Autodesk Fusion 360 part; units mm, degrees
(part 2 of 7)
  spline S17 degree 5 poles (31.8463, -21.6348) (31.8387, -21.6182) (31.8236, -21.585) (31.8007, -21.5353) (31.7701, -21.4693) (31.7314, -21.387) (31.6925, -21.3049) (31.6532, -21.2232) (31.6135, -21.1418) (31.5736, -21.0606) (31.5333, -20.9798) (31.4926, -20.8992) (31.4516, -20.8189) (31.4103, -20.739) (31.3687, -20.6594) (31.3267, -20.58) (31.2844, -20.501) (31.2417, -20.4223) (31.1987, -20.3439) (31.1553, -20.2659) (31.1116, -20.1882) (31.0676, -20.1108) (31.0232, -20.0337) (30.9785, -19.957) (30.9334, -19.8806) (30.888, -19.8046) (30.8422, -19.7289) (30.796, -19.6536) (30.7496, -19.5787) (30.7027, -19.5041) (30.6555, -19.4299) (30.608, -19.356) (30.5601, -19.2825) (30.5118, -19.2094) (30.4631, -19.1368) (30.4141, -19.0645) (30.3647, -18.9925) (30.315, -18.921) (30.2649, -18.85) (30.2144, -18.7793) (30.1635, -18.709) (30.1123, -18.6392) (30.0606, -18.5699) (30.0086, -18.5009) (29.9561, -18.4325) (29.9033, -18.3645) (29.8501, -18.297) (29.7965, -18.2299) (29.7425, -18.1633) (29.6881, -18.0972) (29.6333, -18.0316) (29.578, -17.9666) (29.5222, -17.9021) (29.466, -17.8383) (29.4094, -17.775) (29.3523, -17.7122) (29.2948, -17.65) (29.2369, -17.5883) (29.1786, -17.5272) (29.1198, -17.4666) (29.0604, -17.4069) (29.0004, -17.348) (28.9396, -17.2901) (28.8782, -17.2332) (28.8162, -17.1772) (28.7537, -17.1217) (28.6909, -17.0668) (28.6278, -17.0123) (28.5642, -16.9585) (28.4998, -16.906) (28.434, -16.8556) (28.3799, -16.8175) (28.3382, -16.7905) (28.3099, -16.7732) (28.2957, -16.7647) knots -1 -1 -1 -1 -1 -1 -0.98571429 -0.97142857 -0.95714286 -0.94285714 -0.92857143 -0.91428571 -0.9 -0.88571429 -0.87142857 -0.85714286 -0.84285714 -0.82857143 -0.81428571 -0.8 -0.78571429 -0.77142857 -0.75714286 -0.74285714 -0.72857143 -0.71428571 -0.7 -0.68571429 -0.67142857 -0.65714286 -0.64285714 -0.62857143 -0.61428571 -0.6 -0.58571429 -0.57142857 -0.55714286 -0.54285714 -0.52857143 -0.51428571 -0.5 -0.48571429 -0.47142857 -0.45714286 -0.44285714 -0.42857143 -0.41428571 -0.4 -0.38571429 -0.37142857 -0.35714286 -0.34285714 -0.32857143 -0.31428571 -0.3 -0.28571429 -0.27142857 -0.25714286 -0.24285714 -0.22857143 -0.21428571 -0.2 -0.18571429 -0.17142857 -0.15714286 -0.14285714 -0.12857143 -0.11428571 -0.1 -0.08571429 -0.07142857 -0.05714286 -0.04285714 -0.02857143 -0.01428571 0 0 0 0 0 0
  line L17 (28.2957, -16.7647) -> (27.7863, -16.4626)
  arc A35 (27.1922, -14.356) -> (27.7863, -16.4626) centre (28.5961, -15.0972) ccw
  arc A36 (27.1922, -14.356) -> (27.5975, -13.5607) centre (0, 0) ccw
  arc A37 (29.6509, -12.8031) -> (27.5975, -13.5607) centre (29.0223, -14.2608) ccw
  line L18 (29.6509, -12.8031) -> (30.1947, -13.0376)
  spline S18 degree 5 poles (30.1947, -13.0376) (30.21, -13.0442) (30.2406, -13.0569) (30.2869, -13.0748) (30.3496, -13.0962) (30.429, -13.1197) (30.5094, -13.141) (30.5903, -13.1608) (30.6714, -13.1798) (30.7528, -13.1984) (30.8344, -13.2163) (30.9162, -13.2335) (30.9983, -13.2498) (31.0808, -13.2649) (31.1637, -13.2788) (31.247, -13.2917) (31.3305, -13.3037) (31.4142, -13.315) (31.4982, -13.3255) (31.5823, -13.3355) (31.6666, -13.3448) (31.7511, -13.3534) (31.8359, -13.3614) (31.9208, -13.3686) (32.0059, -13.3751) (32.0911, -13.3809) (32.1766, -13.3861) (32.2622, -13.3906) (32.348, -13.3946) (32.4339, -13.3979) (32.52, -13.4007) (32.6062, -13.4029) (32.6925, -13.4045) (32.779, -13.4055) (32.8656, -13.4059) (32.9523, -13.4058) (33.0392, -13.4051) (33.1262, -13.4038) (33.2132, -13.4021) (33.3004, -13.3997) (33.3877, -13.3969) (33.4751, -13.3935) (33.5626, -13.3896) (33.6502, -13.3852) (33.7379, -13.3803) (33.8257, -13.3748) (33.9136, -13.3689) (34.0016, -13.3624) (34.0896, -13.3555) (34.1778, -13.348) (34.266, -13.3401) (34.3542, -13.3317) (34.4426, -13.3228) (34.531, -13.3134) (34.6195, -13.3035) (34.7081, -13.2932) (34.7967, -13.2824) (34.8854, -13.2711) (34.9741, -13.2594) (35.063, -13.2472) (35.1518, -13.2345) (35.2407, -13.2214) (35.3297, -13.2078) (35.4187, -13.1938) (35.5078, -13.1793) (35.5969, -13.1644) (35.686, -13.1491) (35.7752, -13.1333) (35.8644, -13.117) (35.9537, -13.1003) (36.043, -13.0832) (36.1145, -13.0692) (36.1681, -13.0584) (36.2038, -13.0512) (36.2217, -13.0476) knots 0 0 0 0 0 0 0.01428571 0.02857143 0.04285714 0.05714286 0.07142857 0.08571429 0.1 0.11428571 0.12857143 0.14285714 0.15714286 0.17142857 0.18571429 0.2 0.21428571 0.22857143 0.24285714 0.25714286 0.27142857 0.28571429 0.3 0.31428571 0.32857143 0.34285714 0.35714286 0.37142857 0.38571429 0.4 0.41428571 0.42857143 0.44285714 0.45714286 0.47142857 0.48571429 0.5 0.51428571 0.52857143 0.54285714 0.55714286 0.57142857 0.58571429 0.6 0.61428571 0.62857143 0.64285714 0.65714286 0.67142857 0.68571429 0.7 0.71428571 0.72857143 0.74285714 0.75714286 0.77142857 0.78571429 0.8 0.81428571 0.82857143 0.84285714 0.85714286 0.87142857 0.88571429 0.9 0.91428571 0.92857143 0.94285714 0.95714286 0.97142857 0.98571429 1 1 1 1 1 1
  arc A38 (36.2217, -13.0476) -> (36.9731, -10.7349) centre (0, 0) ccw
  spline S19 degree 5 poles (36.9731, -10.7349) (36.9608, -10.7214) (36.9361, -10.6946) (36.8991, -10.6544) (36.8495, -10.601) (36.7873, -10.5347) (36.7249, -10.4687) (36.6623, -10.4031) (36.5994, -10.3379) (36.5363, -10.2731) (36.473, -10.2086) (36.4095, -10.1446) (36.3457, -10.0809) (36.2817, -10.0176) (36.2175, -9.9548) (36.153, -9.8923) (36.0883, -9.8302) (36.0235, -9.7686) (35.9583, -9.7073) (35.893, -9.6465) (35.8274, -9.5861) (35.7616, -9.5261) (35.6956, -9.4665) (35.6293, -9.4074) (35.5629, -9.3487) (35.4962, -9.2904) (35.4292, -9.2326) (35.3621, -9.1752) (35.2947, -9.1183) (35.2271, -9.0618) (35.1593, -9.0058) (35.0912, -8.9503) (35.023, -8.8952) (34.9545, -8.8406) (34.8857, -8.7865) (34.8168, -8.7329) (34.7476, -8.6798) (34.6782, -8.6271) (34.6086, -8.575) (34.5387, -8.5234) (34.4686, -8.4723) (34.3983, -8.4218) (34.3277, -8.3717) (34.257, -8.3223) (34.1859, -8.2734) (34.1147, -8.225) (34.0432, -8.1773) (33.9715, -8.13) (33.8996, -8.0834) (33.8274, -8.0373) (33.755, -7.9919) (33.6823, -7.9471) (33.6094, -7.9031) (33.5362, -7.8597) (33.4627, -7.817) (33.389, -7.775) (33.3151, -7.7336) (33.241, -7.6928) (33.1666, -7.6526) (33.092, -7.6133) (33.0171, -7.5748) (32.9418, -7.5373) (32.8662, -7.5011) (32.7902, -7.4659) (32.7139, -7.4318) (32.6373, -7.3983) (32.5606, -7.3655) (32.4838, -7.3332) (32.4067, -7.3017) (32.3292, -7.2716) (32.251, -7.244) (32.1878, -7.2245) (32.1398, -7.2117) (32.1076, -7.204) (32.0914, -7.2004) knots -1 -1 -1 -1 -1 -1 -0.98571429 -0.97142857 -0.95714286 -0.94285714 -0.92857143 -0.91428571 -0.9 -0.88571429 -0.87142857 -0.85714286 -0.84285714 -0.82857143 -0.81428571 -0.8 -0.78571429 -0.77142857 -0.75714286 -0.74285714 -0.72857143 -0.71428571 -0.7 -0.68571429 -0.67142857 -0.65714286 -0.64285714 -0.62857143 -0.61428571 -0.6 -0.58571429 -0.57142857 -0.55714286 -0.54285714 -0.52857143 -0.51428571 -0.5 -0.48571429 -0.47142857 -0.45714286 -0.44285714 -0.42857143 -0.41428571 -0.4 -0.38571429 -0.37142857 -0.35714286 -0.34285714 -0.32857143 -0.31428571 -0.3 -0.28571429 -0.27142857 -0.25714286 -0.24285714 -0.22857143 -0.21428571 -0.2 -0.18571429 -0.17142857 -0.15714286 -0.14285714 -0.12857143 -0.11428571 -0.1 -0.08571429 -0.07142857 -0.05714286 -0.04285714 -0.02857143 -0.01428571 0 0 0 0 0 0
  line L19 (32.0914, -7.2004) -> (31.5136, -7.0705)
  arc A39 (30.2976, -5.2505) -> (31.5136, -7.0705) centre (31.8618, -5.5216) ccw
  arc A40 (30.2976, -5.2505) -> (30.4372, -4.3689) centre (0, 0) ccw
  arc A41 (32.1561, -3.0138) -> (30.4372, -4.3689) centre (32.0086, -4.5945) ccw
  line L20 (32.1561, -3.0138) -> (32.7458, -3.0688)
  spline S20 degree 5 poles (32.7458, -3.0688) (32.7623, -3.0704) (32.7953, -3.073) (32.8449, -3.0757) (32.9111, -3.0767) (32.994, -3.0745) (33.0769, -3.0699) (33.16, -3.0638) (33.2431, -3.0568) (33.3262, -3.0493) (33.4093, -3.0411) (33.4924, -3.0322) (33.5756, -3.0223) (33.6587, -3.0111) (33.7419, -2.9988) (33.825, -2.9854) (33.9081, -2.971) (33.9913, -2.9558) (34.0744, -2.9399) (34.1575, -2.9233) (34.2405, -2.9061) (34.3236, -2.8882) (34.4066, -2.8696) (34.4896, -2.8502) (34.5725, -2.8301) (34.6554, -2.8093) (34.7383, -2.7878) (34.8211, -2.7657) (34.9039, -2.7429) (34.9867, -2.7195) (35.0694, -2.6956) (35.152, -2.671) (35.2346, -2.6459) (35.3172, -2.6201) (35.3997, -2.5937) (35.4821, -2.5668) (35.5645, -2.5393) (35.6469, -2.5113) (35.7291, -2.4827) (35.8113, -2.4535) (35.8935, -2.4238) (35.9756, -2.3936) (36.0576, -2.3629) (36.1395, -2.3316) (36.2214, -2.2998) (36.3032, -2.2675) (36.385, -2.2347) (36.4666, -2.2013) (36.5482, -2.1675) (36.6297, -2.1332) (36.7112, -2.0984) (36.7925, -2.0631) (36.8738, -2.0274) (36.955, -1.9911) (37.0361, -1.9544) (37.1172, -1.9172) (37.1981, -1.8795) (37.279, -1.8414) (37.3598, -1.8028) (37.4405, -1.7638) (37.5211, -1.7243) (37.6016, -1.6843) (37.682, -1.6439) (37.7623, -1.6031) (37.8425, -1.5618) (37.9227, -1.5201) (38.0027, -1.4779) (38.0826, -1.4353) (38.1625, -1.3923) (38.2422, -1.3489) (38.3218, -1.305) (38.3855, -1.2695) (38.4332, -1.2428) (38.4649, -1.2248) (38.4808, -1.2158) knots 0 0 0 0 0 0 0.01428571 0.02857143 0.04285714 0.05714286 0.07142857 0.08571429 0.1 0.11428571 0.12857143 0.14285714 0.15714286 0.17142857 0.18571429 0.2 0.21428571 0.22857143 0.24285714 0.25714286 0.27142857 0.28571429 0.3 0.31428571 0.32857143 0.34285714 0.35714286 0.37142857 0.38571429 0.4 0.41428571 0.42857143 0.44285714 0.45714286 0.47142857 0.48571429 0.5 0.51428571 0.52857143 0.54285714 0.55714286 0.57142857 0.58571429 0.6 0.61428571 0.62857143 0.64285714 0.65714286 0.67142857 0.68571429 0.7 0.71428571 0.72857143 0.74285714 0.75714286 0.77142857 0.78571429 0.8 0.81428571 0.82857143 0.84285714 0.85714286 0.87142857 0.88571429 0.9 0.91428571 0.92857143 0.94285714 0.95714286 0.97142857 0.98571429 1 1 1 1 1 1
  arc A42 (38.4808, -1.2158) -> (38.4808, 1.2158) centre (0, 0) ccw
  spline S21 degree 5 poles (38.4808, 1.2158) (38.4649, 1.2248) (38.4332, 1.2428) (38.3855, 1.2695) (38.3218, 1.305) (38.2422, 1.3489) (38.1625, 1.3923) (38.0826, 1.4353) (38.0027, 1.4779) (37.9227, 1.5201) (37.8425, 1.5618) (37.7623, 1.6031) (37.682, 1.6439) (37.6016, 1.6843) (37.5211, 1.7243) (37.4405, 1.7638) (37.3598, 1.8028) (37.279, 1.8414) (37.1981, 1.8795) (37.1172, 1.9172) (37.0361, 1.9544) (36.955, 1.9911) (36.8738, 2.0274) (36.7925, 2.0631) (36.7112, 2.0984) (36.6297, 2.1332) (36.5482, 2.1675) (36.4666, 2.2013) (36.385, 2.2347) (36.3032, 2.2675) (36.2214, 2.2998) (36.1395, 2.3316) (36.0576, 2.3629) (35.9756, 2.3936) (35.8935, 2.4238) (35.8113, 2.4535) (35.7291, 2.4827) (35.6469, 2.5113) (35.5645, 2.5393) (35.4821, 2.5668) (35.3997, 2.5937) (35.3172, 2.6201) (35.2346, 2.6459) (35.152, 2.671) (35.0694, 2.6956) (34.9867, 2.7195) (34.9039, 2.7429) (34.8211, 2.7657) (34.7383, 2.7878) (34.6554, 2.8093) (34.5725, 2.8301) (34.4896, 2.8502) (34.4066, 2.8696) (34.3236, 2.8882) (34.2405, 2.9061) (34.1575, 2.9233) (34.0744, 2.9399) (33.9913, 2.9558) (33.9081, 2.971) (33.825, 2.9854) (33.7419, 2.9988) (33.6587, 3.0111) (33.5756, 3.0223) (33.4924, 3.0322) (33.4093, 3.0411) (33.3262, 3.0493) (33.2431, 3.0568) (33.16, 3.0638) (33.0769, 3.0699) (32.994, 3.0745) (32.9111, 3.0767) (32.8449, 3.0757) (32.7953, 3.073) (32.7623, 3.0704) (32.7458, 3.0688) knots -1 -1 -1 -1 -1 -1 -0.98571429 -0.97142857 -0.95714286 -0.94285714 -0.92857143 -0.91428571 -0.9 -0.88571429 -0.87142857 -0.85714286 -0.84285714 -0.82857143 -0.81428571 -0.8 -0.78571429 -0.77142857 -0.75714286 -0.74285714 -0.72857143 -0.71428571 -0.7 -0.68571429 -0.67142857 -0.65714286 -0.64285714 -0.62857143 -0.61428571 -0.6 -0.58571429 -0.57142857 -0.55714286 -0.54285714 -0.52857143 -0.51428571 -0.5 -0.48571429 -0.47142857 -0.45714286 -0.44285714 -0.42857143 -0.41428571 -0.4 -0.38571429 -0.37142857 -0.35714286 -0.34285714 -0.32857143 -0.31428571 -0.3 -0.28571429 -0.27142857 -0.25714286 -0.24285714 -0.22857143 -0.21428571 -0.2 -0.18571429 -0.17142857 -0.15714286 -0.14285714 -0.12857143 -0.11428571 -0.1 -0.08571429 -0.07142857 -0.05714286 -0.04285714 -0.02857143 -0.01428571 0 0 0 0 0 0
  line L21 (32.7458, 3.0688) -> (32.1561, 3.0138)
  arc A43 (30.4372, 4.3689) -> (32.1561, 3.0138) centre (32.0086, 4.5945) ccw
  arc A44 (30.4372, 4.3689) -> (30.2976, 5.2505) centre (0, 0) ccw
  arc A45 (31.5136, 7.0705) -> (30.2976, 5.2505) centre (31.8618, 5.5216) ccw
  line L22 (31.5136, 7.0705) -> (32.0914, 7.2004)
  spline S22 degree 5 poles (32.0914, 7.2004) (32.1076, 7.204) (32.1398, 7.2117) (32.1878, 7.2245) (32.251, 7.244) (32.3292, 7.2716) (32.4067, 7.3017) (32.4838, 7.3332) (32.5606, 7.3655) (32.6373, 7.3983) (32.7139, 7.4318) (32.7902, 7.4659) (32.8662, 7.5011) (32.9418, 7.5373) (33.0171, 7.5748) (33.092, 7.6133) (33.1666, 7.6526) (33.241, 7.6928) (33.3151, 7.7336) (33.389, 7.775) (33.4627, 7.817) (33.5362, 7.8597) (33.6094, 7.9031) (33.6823, 7.9471) (33.755, 7.9919) (33.8274, 8.0373) (33.8996, 8.0834) (33.9715, 8.13) (34.0432, 8.1773) (34.1147, 8.225) (34.1859, 8.2734) (34.257, 8.3223) (34.3277, 8.3717) (34.3983, 8.4218) (34.4686, 8.4723) (34.5387, 8.5234) (34.6086, 8.575) (34.6782, 8.6271) (34.7476, 8.6798) (34.8168, 8.7329) (34.8857, 8.7865) (34.9545, 8.8406) (35.023, 8.8952) (35.0912, 8.9503) (35.1593, 9.0058) (35.2271, 9.0618) (35.2947, 9.1183) (35.3621, 9.1752) (35.4292, 9.2326) (35.4962, 9.2904) (35.5629, 9.3487) (35.6293, 9.4074) (35.6956, 9.4665) (35.7616, 9.5261) (35.8274, 9.5861) (35.893, 9.6465) (35.9583, 9.7073) (36.0235, 9.7686) (36.0883, 9.8302) (36.153, 9.8923) (36.2175, 9.9548) (36.2817, 10.0176) (36.3457, 10.0809) (36.4095, 10.1446) (36.473, 10.2086) (36.5363, 10.2731) (36.5994, 10.3379) (36.6623, 10.4031) (36.7249, 10.4687) (36.7873, 10.5347) (36.8495, 10.601) (36.8991, 10.6544) (36.9361, 10.6946) (36.9608, 10.7214) (36.9731, 10.7349) knots 0 0 0 0 0 0 0.01428571 0.02857143 0.04285714 0.05714286 0.07142857 0.08571429 0.1 0.11428571 0.12857143 0.14285714 0.15714286 0.17142857 0.18571429 0.2 0.21428571 0.22857143 0.24285714 0.25714286 0.27142857 0.28571429 0.3 0.31428571 0.32857143 0.34285714 0.35714286 0.37142857 0.38571429 0.4 0.41428571 0.42857143 0.44285714 0.45714286 0.47142857 0.48571429 0.5 0.51428571 0.52857143 0.54285714 0.55714286 0.57142857 0.58571429 0.6 0.61428571 0.62857143 0.64285714 0.65714286 0.67142857 0.68571429 0.7 0.71428571 0.72857143 0.74285714 0.75714286 0.77142857 0.78571429 0.8 0.81428571 0.82857143 0.84285714 0.85714286 0.87142857 0.88571429 0.9 0.91428571 0.92857143 0.94285714 0.95714286 0.97142857 0.98571429 1 1 1 1 1 1
  arc A46 (36.9731, 10.7349) -> (36.2217, 13.0476) centre (0, 0) ccw
  spline S23 degree 5 poles (36.2217, 13.0476) (36.2038, 13.0512) (36.1681, 13.0584) (36.1145, 13.0692) (36.043, 13.0832) (35.9537, 13.1003) (35.8644, 13.117) (35.7752, 13.1333) (35.686, 13.1491) (35.5969, 13.1644) (35.5078, 13.1793) (35.4187, 13.1938) (35.3297, 13.2078) (35.2407, 13.2214) (35.1518, 13.2345) (35.063, 13.2472) (34.9741, 13.2594) (34.8854, 13.2711) (34.7967, 13.2824) (34.7081, 13.2932) (34.6195, 13.3035) (34.531, 13.3134) (34.4426, 13.3228) (34.3542, 13.3317) (34.266, 13.3401) (34.1778, 13.348) (34.0896, 13.3555) (34.0016, 13.3624) (33.9136, 13.3689) (33.8257, 13.3748) (33.7379, 13.3803) (33.6502, 13.3852) (33.5626, 13.3896) (33.4751, 13.3935) (33.3877, 13.3969) (33.3004, 13.3997) (33.2132, 13.4021) (33.1262, 13.4038) (33.0392, 13.4051) (32.9523, 13.4058) (32.8656, 13.4059) (32.779, 13.4055) (32.6925, 13.4045) (32.6062, 13.4029) (32.52, 13.4007) (32.4339, 13.3979) (32.348, 13.3946) (32.2622, 13.3906) (32.1766, 13.3861) (32.0911, 13.3809) (32.0059, 13.3751) (31.9208, 13.3686) (31.8359, 13.3614) (31.7511, 13.3534) (31.6666, 13.3448) (31.5823, 13.3355) (31.4982, 13.3255) (31.4142, 13.315) (31.3305, 13.3037) (31.247, 13.2917) (31.1637, 13.2788) (31.0808, 13.2649) (30.9983, 13.2498) (30.9162, 13.2335) (30.8344, 13.2163) (30.7528, 13.1984) (30.6714, 13.1798) (30.5903, 13.1608) (30.5094, 13.141) (30.429, 13.1197) (30.3496, 13.0962) (30.2869, 13.0748) (30.2406, 13.0569) (30.21, 13.0442) (30.1947, 13.0376) knots -1 -1 -1 -1 -1 -1 -0.98571429 -0.97142857 -0.95714286 -0.94285714 -0.92857143 -0.91428571 -0.9 -0.88571429 -0.87142857 -0.85714286 -0.84285714 -0.82857143 -0.81428571 -0.8 -0.78571429 -0.77142857 -0.75714286 -0.74285714 -0.72857143 -0.71428571 -0.7 -0.68571429 -0.67142857 -0.65714286 -0.64285714 -0.62857143 -0.61428571 -0.6 -0.58571429 -0.57142857 -0.55714286 -0.54285714 -0.52857143 -0.51428571 -0.5 -0.48571429 -0.47142857 -0.45714286 -0.44285714 -0.42857143 -0.41428571 -0.4 -0.38571429 -0.37142857 -0.35714286 -0.34285714 -0.32857143 -0.31428571 -0.3 -0.28571429 -0.27142857 -0.25714286 -0.24285714 -0.22857143 -0.21428571 -0.2 -0.18571429 -0.17142857 -0.15714286 -0.14285714 -0.12857143 -0.11428571 -0.1 -0.08571429 -0.07142857 -0.05714286 -0.04285714 -0.02857143 -0.01428571 0 0 0 0 0 0
  line L23 (30.1947, 13.0376) -> (29.6509, 12.8031)
  arc A47 (27.5975, 13.5607) -> (29.6509, 12.8031) centre (29.0223, 14.2608) ccw
  arc A48 (27.5975, 13.5607) -> (27.1922, 14.356) centre (0, 0) ccw
  arc A49 (27.7863, 16.4626) -> (27.1922, 14.356) centre (28.5961, 15.0972) ccw
  line L24 (27.7863, 16.4626) -> (28.2957, 16.7647)
  spline S24 degree 5 poles (28.2957, 16.7647) (28.3099, 16.7732) (28.3382, 16.7905) (28.3799, 16.8175) (28.434, 16.8556) (28.4998, 16.906) (28.5642, 16.9585) (28.6278, 17.0123) (28.6909, 17.0668) (28.7537, 17.1217) (28.8162, 17.1772) (28.8782, 17.2332) (28.9396, 17.2901) (29.0004, 17.348) (29.0604, 17.4069) (29.1198, 17.4666) (29.1786, 17.5272) (29.2369, 17.5883) (29.2948, 17.65) (29.3523, 17.7122) (29.4094, 17.775) (29.466, 17.8383) (29.5222, 17.9021) (29.578, 17.9666) (29.6333, 18.0316) (29.6881, 18.0972) (29.7425, 18.1633) (29.7965, 18.2299) (29.8501, 18.297) (29.9033, 18.3645) (29.9561, 18.4325) (30.0086, 18.5009) (30.0606, 18.5699) (30.1123, 18.6392) (30.1635, 18.709) (30.2144, 18.7793) (30.2649, 18.85) (30.315, 18.921) (30.3647, 18.9925) (30.4141, 19.0645) (30.4631, 19.1368) (30.5118, 19.2094) (30.5601, 19.2825) (30.608, 19.356) (30.6555, 19.4299) (30.7027, 19.5041) (30.7496, 19.5787) (30.796, 19.6536) (30.8422, 19.7289) (30.888, 19.8046) (30.9334, 19.8806) (30.9785, 19.957) (31.0232, 20.0337) (31.0676, 20.1108) (31.1116, 20.1882) (31.1553, 20.2659) (31.1987, 20.3439) (31.2417, 20.4223) (31.2844, 20.501) (31.3267, 20.58) (31.3687, 20.6594) (31.4103, 20.739) (31.4516, 20.8189) (31.4926, 20.8992) (31.5333, 20.9798) (31.5736, 21.0606) (31.6135, 21.1418) (31.6532, 21.2232) (31.6925, 21.3049) (31.7314, 21.387) (31.7701, 21.4693) (31.8007, 21.5353) (31.8236, 21.585) (31.8387, 21.6182) (31.8463, 21.6348) knots 0 0 0 0 0 0 0.01428571 0.02857143 0.04285714 0.05714286 0.07142857 0.08571429 0.1 0.11428571 0.12857143 0.14285714 0.15714286 0.17142857 0.18571429 0.2 0.21428571 0.22857143 0.24285714 0.25714286 0.27142857 0.28571429 0.3 0.31428571 0.32857143 0.34285714 0.35714286 0.37142857 0.38571429 0.4 0.41428571 0.42857143 0.44285714 0.45714286 0.47142857 0.48571429 0.5 0.51428571 0.52857143 0.54285714 0.55714286 0.57142857 0.58571429 0.6 0.61428571 0.62857143 0.64285714 0.65714286 0.67142857 0.68571429 0.7 0.71428571 0.72857143 0.74285714 0.75714286 0.77142857 0.78571429 0.8 0.81428571 0.82857143 0.84285714 0.85714286 0.87142857 0.88571429 0.9 0.91428571 0.92857143 0.94285714 0.95714286 0.97142857 0.98571429 1 1 1 1 1 1
  arc A50 (31.8463, 21.6348) -> (30.417, 23.6021) centre (0, 0) ccw
  spline S25 degree 5 poles (30.417, 23.6021) (30.3988, 23.6) (30.3626, 23.5959) (30.3083, 23.5895) (30.236, 23.5808) (30.1458, 23.5695) (30.0557, 23.5577) (29.9658, 23.5456) (29.8761, 23.5331) (29.7866, 23.5201) (29.6972, 23.5068) (29.6081, 23.493) (29.5191, 23.4789) (29.4303, 23.4643) (29.3417, 23.4493) (29.2532, 23.4339) (29.165, 23.418) (29.077, 23.4018) (28.9892, 23.3851) (28.9015, 23.368) (28.8141, 23.3504) (28.7269, 23.3325) (28.6399, 23.3141) (28.5531, 23.2952) (28.4666, 23.2759) (28.3802, 23.2562) (28.2941, 23.2361) (28.2082, 23.2155) (28.1226, 23.1944) (28.0371, 23.1729) (27.952, 23.151) (27.867, 23.1286) (27.7824, 23.1057) (27.6979, 23.0824) (27.6138, 23.0586) (27.5298, 23.0343) (27.4462, 23.0096) (27.3628, 22.9844) (27.2797, 22.9587) (27.1969, 22.9325) (27.1144, 22.9058) (27.0322, 22.8786) (26.9502, 22.8509) (26.8686, 22.8227) (26.7873, 22.794) (26.7063, 22.7648) (26.6256, 22.7351) (26.5453, 22.7048) (26.4652, 22.674) (26.3856, 22.6427) (26.3062, 22.6108) (26.2273, 22.5783) (26.1488, 22.5452) (26.0707, 22.5115) (25.993, 22.4772) (25.9157, 22.4423) (25.8387, 22.4068) (25.7622, 22.3708) (25.686, 22.3343) (25.6103, 22.297) (25.5351, 22.259) (25.4606, 22.2202) (25.3867, 22.1803) (25.3136, 22.1395) (25.2411, 22.0978) (25.1691, 22.0555) (25.0975, 22.0128) (25.0261, 21.9696) (24.9554, 21.9257) (24.8855, 21.8807) (24.8172, 21.8337) (24.7642, 21.794) (24.7257, 21.7627) (24.7005, 21.7412) (24.6881, 21.7302) knots -1 -1 -1 -1 -1 -1 -0.98571429 -0.97142857 -0.95714286 -0.94285714 -0.92857143 -0.91428571 -0.9 -0.88571429 -0.87142857 -0.85714286 -0.84285714 -0.82857143 -0.81428571 -0.8 -0.78571429 -0.77142857 -0.75714286 -0.74285714 -0.72857143 -0.71428571 -0.7 -0.68571429 -0.67142857 -0.65714286 -0.64285714 -0.62857143 -0.61428571 -0.6 -0.58571429 -0.57142857 -0.55714286 -0.54285714 -0.52857143 -0.51428571 -0.5 -0.48571429 -0.47142857 -0.45714286 -0.44285714 -0.42857143 -0.41428571 -0.4 -0.38571429 -0.37142857 -0.35714286 -0.34285714 -0.32857143 -0.31428571 -0.3 -0.28571429 -0.27142857 -0.25714286 -0.24285714 -0.22857143 -0.21428571 -0.2 -0.18571429 -0.17142857 -0.15714286 -0.14285714 -0.12857143 -0.11428571 -0.1 -0.08571429 -0.07142857 -0.05714286 -0.04285714 -0.02857143 -0.01428571 0 0 0 0 0 0
  line L25 (24.6881, 21.7302) -> (24.2433, 21.3391)
  arc A51 (22.0563, 21.4251) -> (24.2433, 21.3391) centre (23.195, 22.5312) ccw
  arc A52 (22.0563, 21.4251) -> (21.4251, 22.0563) centre (0, 0) ccw
  arc A53 (21.3391, 24.2433) -> (21.4251, 22.0563) centre (22.5312, 23.195) ccw
  line L26 (21.3391, 24.2433) -> (21.7302, 24.6881)
  spline S26 degree 5 poles (21.7302, 24.6881) (21.7412, 24.7005) (21.7627, 24.7257) (21.794, 24.7642) (21.8337, 24.8172) (21.8807, 24.8855) (21.9257, 24.9554) (21.9696, 25.0261) (22.0128, 25.0975) (22.0555, 25.1691) (22.0978, 25.2411) (22.1395, 25.3136) (22.1803, 25.3867) (22.2202, 25.4606) (22.259, 25.5351) (22.297, 25.6103) (22.3343, 25.686) (22.3708, 25.7622) (22.4068, 25.8387) (22.4423, 25.9157) (22.4772, 25.993) (22.5115, 26.0707) (22.5452, 26.1488) (22.5783, 26.2273) (22.6108, 26.3062) (22.6427, 26.3856) (22.674, 26.4652) (22.7048, 26.5453) (22.7351, 26.6256) (22.7648, 26.7063) (22.794, 26.7873) (22.8227, 26.8686) (22.8509, 26.9502) (22.8786, 27.0322) (22.9058, 27.1144) (22.9325, 27.1969) (22.9587, 27.2797) (22.9844, 27.3628) (23.0096, 27.4462) (23.0343, 27.5298) (23.0586, 27.6138) (23.0824, 27.6979) (23.1057, 27.7824) (23.1286, 27.867) (23.151, 27.952) (23.1729, 28.0371) (23.1944, 28.1226) (23.2155, 28.2082) (23.2361, 28.2941) (23.2562, 28.3802) (23.2759, 28.4666) (23.2952, 28.5531) (23.3141, 28.6399) (23.3325, 28.7269) (23.3504, 28.8141) (23.368, 28.9015) (23.3851, 28.9892) (23.4018, 29.077) (23.418, 29.165) (23.4339, 29.2532) (23.4493, 29.3417) (23.4643, 29.4303) (23.4789, 29.5191) (23.493, 29.6081) (23.5068, 29.6972) (23.5201, 29.7866) (23.5331, 29.8761) (23.5456, 29.9658) (23.5577, 30.0557) (23.5695, 30.1458) (23.5808, 30.236) (23.5895, 30.3083) (23.5959, 30.3626) (23.6, 30.3988) (23.6021, 30.417) knots 0 0 0 0 0 0 0.01428571 0.02857143 0.04285714 0.05714286 0.07142857 0.08571429 0.1 0.11428571 0.12857143 0.14285714 0.15714286 0.17142857 0.18571429 0.2 0.21428571 0.22857143 0.24285714 0.25714286 0.27142857 0.28571429 0.3 0.31428571 0.32857143 0.34285714 0.35714286 0.37142857 0.38571429 0.4 0.41428571 0.42857143 0.44285714 0.45714286 0.47142857 0.48571429 0.5 0.51428571 0.52857143 0.54285714 0.55714286 0.57142857 0.58571429 0.6 0.61428571 0.62857143 0.64285714 0.65714286 0.67142857 0.68571429 0.7 0.71428571 0.72857143 0.74285714 0.75714286 0.77142857 0.78571429 0.8 0.81428571 0.82857143 0.84285714 0.85714286 0.87142857 0.88571429 0.9 0.91428571 0.92857143 0.94285714 0.95714286 0.97142857 0.98571429 1 1 1 1 1 1
  arc A54 (23.6021, 30.417) -> (21.6348, 31.8463) centre (0, 0) ccw
  spline S27 degree 5 poles (21.6348, 31.8463) (21.6182, 31.8387) (21.585, 31.8236) (21.5353, 31.8007) (21.4693, 31.7701) (21.387, 31.7314) (21.3049, 31.6925) (21.2232, 31.6532) (21.1418, 31.6135) (21.0606, 31.5736) (20.9798, 31.5333) (20.8992, 31.4926) (20.8189, 31.4516) (20.739, 31.4103) (20.6594, 31.3687) (20.58, 31.3267) (20.501, 31.2844) (20.4223, 31.2417) (20.3439, 31.1987) (20.2659, 31.1553) (20.1882, 31.1116) (20.1108, 31.0676) (20.0337, 31.0232) (19.957, 30.9785) (19.8806, 30.9334) (19.8046, 30.888) (19.7289, 30.8422) (19.6536, 30.796) (19.5787, 30.7496) (19.5041, 30.7027) (19.4299, 30.6555) (19.356, 30.608) (19.2825, 30.5601) (19.2094, 30.5118) (19.1368, 30.4631) (19.0645, 30.4141) (18.9925, 30.3647) (18.921, 30.315) (18.85, 30.2649) (18.7793, 30.2144) (18.709, 30.1635) (18.6392, 30.1123) (18.5699, 30.0606) (18.5009, 30.0086) (18.4325, 29.9561) (18.3645, 29.9033) (18.297, 29.8501) (18.2299, 29.7965) (18.1633, 29.7425) (18.0972, 29.6881) (18.0316, 29.6333) (17.9666, 29.578) (17.9021, 29.5222) (17.8383, 29.466) (17.775, 29.4094) (17.7122, 29.3523) (17.65, 29.2948) (17.5883, 29.2369) (17.5272, 29.1786) (17.4666, 29.1198) (17.4069, 29.0604) (17.348, 29.0004) (17.2901, 28.9396) (17.2332, 28.8782) (17.1772, 28.8162) (17.1217, 28.7537) (17.0668, 28.6909) (17.0123, 28.6278) (16.9585, 28.5642) (16.906, 28.4998) (16.8556, 28.434) (16.8175, 28.3799) (16.7905, 28.3382) (16.7732, 28.3099) (16.7647, 28.2957) knots -1 -1 -1 -1 -1 -1 -0.98571429 -0.97142857 -0.95714286 -0.94285714 -0.92857143 -0.91428571 -0.9 -0.88571429 -0.87142857 -0.85714286 -0.84285714 -0.82857143 -0.81428571 -0.8 -0.78571429 -0.77142857 -0.75714286 -0.74285714 -0.72857143 -0.71428571 -0.7 -0.68571429 -0.67142857 -0.65714286 -0.64285714 -0.62857143 -0.61428571 -0.6 -0.58571429 -0.57142857 -0.55714286 -0.54285714 -0.52857143 -0.51428571 -0.5 -0.48571429 -0.47142857 -0.45714286 -0.44285714 -0.42857143 -0.41428571 -0.4 -0.38571429 -0.37142857 -0.35714286 -0.34285714 -0.32857143 -0.31428571 -0.3 -0.28571429 -0.27142857 -0.25714286 -0.24285714 -0.22857143 -0.21428571 -0.2 -0.18571429 -0.17142857 -0.15714286 -0.14285714 -0.12857143 -0.11428571 -0.1 -0.08571429 -0.07142857 -0.05714286 -0.04285714 -0.02857143 -0.01428571 0 0 0 0 0 0
  line L27 (16.7647, 28.2957) -> (16.4626, 27.7863)
  arc A55 (14.356, 27.1922) -> (16.4626, 27.7863) centre (15.0972, 28.5961) ccw
  arc A56 (14.356, 27.1922) -> (13.5607, 27.5975) centre (0, 0) ccw
  arc A57 (12.8031, 29.6509) -> (13.5607, 27.5975) centre (14.2608, 29.0223) ccw
  line L28 (12.8031, 29.6509) -> (13.0376, 30.1947)
  spline S28 degree 5 poles (13.0376, 30.1947) (13.0442, 30.21) (13.0569, 30.2406) (13.0748, 30.2869) (13.0962, 30.3496) (13.1197, 30.429) (13.141, 30.5094) (13.1608, 30.5903) (13.1798, 30.6714) (13.1984, 30.7528) (13.2163, 30.8344) (13.2335, 30.9162) (13.2498, 30.9983) (13.2649, 31.0808) (13.2788, 31.1637) (13.2917, 31.247) (13.3037, 31.3305) (13.315, 31.4142) (13.3255, 31.4982) (13.3355, 31.5823) (13.3448, 31.6666) (13.3534, 31.7511) (13.3614, 31.8359) (13.3686, 31.9208) (13.3751, 32.0059) (13.3809, 32.0911) (13.3861, 32.1766) (13.3906, 32.2622) (13.3946, 32.348) (13.3979, 32.4339) (13.4007, 32.52) (13.4029, 32.6062) (13.4045, 32.6925) (13.4055, 32.779) (13.4059, 32.8656) (13.4058, 32.9523) (13.4051, 33.0392) (13.4038, 33.1262) (13.4021, 33.2132) (13.3997, 33.3004) (13.3969, 33.3877) (13.3935, 33.4751) (13.3896, 33.5626) (13.3852, 33.6502) (13.3803, 33.7379) (13.3748, 33.8257) (13.3689, 33.9136) (13.3624, 34.0016) (13.3555, 34.0896) (13.348, 34.1778) (13.3401, 34.266) (13.3317, 34.3542) (13.3228, 34.4426) (13.3134, 34.531) (13.3035, 34.6195) (13.2932, 34.7081) (13.2824, 34.7967) (13.2711, 34.8854) (13.2594, 34.9741) (13.2472, 35.063) (13.2345, 35.1518) (13.2214, 35.2407) (13.2078, 35.3297) (13.1938, 35.4187) (13.1793, 35.5078) (13.1644, 35.5969) (13.1491, 35.686) (13.1333, 35.7752) (13.117, 35.8644) (13.1003, 35.9537) (13.0832, 36.043) (13.0692, 36.1145) (13.0584, 36.1681) (13.0512, 36.2038) (13.0476, 36.2217) knots 0 0 0 0 0 0 0.01428571 0.02857143 0.04285714 0.05714286 0.07142857 0.08571429 0.1 0.11428571 0.12857143 0.14285714 0.15714286 0.17142857 0.18571429 0.2 0.21428571 0.22857143 0.24285714 0.25714286 0.27142857 0.28571429 0.3 0.31428571 0.32857143 0.34285714 0.35714286 0.37142857 0.38571429 0.4 0.41428571 0.42857143 0.44285714 0.45714286 0.47142857 0.48571429 0.5 0.51428571 0.52857143 0.54285714 0.55714286 0.57142857 0.58571429 0.6 0.61428571 0.62857143 0.64285714 0.65714286 0.67142857 0.68571429 0.7 0.71428571 0.72857143 0.74285714 0.75714286 0.77142857 0.78571429 0.8 0.81428571 0.82857143 0.84285714 0.85714286 0.87142857 0.88571429 0.9 0.91428571 0.92857143 0.94285714 0.95714286 0.97142857 0.98571429 1 1 1 1 1 1
  arc A58 (13.0476, 36.2217) -> (10.7349, 36.9731) centre (0, 0) ccw
  spline S29 degree 5 poles (10.7349, 36.9731) (10.7214, 36.9608) (10.6946, 36.9361) (10.6544, 36.8991) (10.601, 36.8495) (10.5347, 36.7873) (10.4687, 36.7249) (10.4031, 36.6623) (10.3379, 36.5994) (10.2731, 36.5363) (10.2086, 36.473) (10.1446, 36.4095) (10.0809, 36.3457) (10.0176, 36.2817) (9.9548, 36.2175) (9.8923, 36.153) (9.8302, 36.0883) (9.7686, 36.0235) (9.7073, 35.9583) (9.6465, 35.893) (9.5861, 35.8274) (9.5261, 35.7616) (9.4665, 35.6956) (9.4074, 35.6293) (9.3487, 35.5629) (9.2904, 35.4962) (9.2326, 35.4292) (9.1752, 35.3621) (9.1183, 35.2947) (9.0618, 35.2271) (9.0058, 35.1593) (8.9503, 35.0912) (8.8952, 35.023) (8.8406, 34.9545) (8.7865, 34.8857) (8.7329, 34.8168) (8.6798, 34.7476) (8.6271, 34.6782) (8.575, 34.6086) (8.5234, 34.5387) (8.4723, 34.4686) (8.4218, 34.3983) (8.3717, 34.3277) (8.3223, 34.257) (8.2734, 34.1859) (8.225, 34.1147) (8.1773, 34.0432) (8.13, 33.9715) (8.0834, 33.8996) (8.0373, 33.8274) (7.9919, 33.755) (7.9471, 33.6823) (7.9031, 33.6094) (7.8597, 33.5362) (7.817, 33.4627) (7.775, 33.389) (7.7336, 33.3151) (7.6928, 33.241) (7.6526, 33.1666) (7.6133, 33.092) (7.5748, 33.0171) (7.5373, 32.9418) (7.5011, 32.8662) (7.4659, 32.7902) (7.4318, 32.7139) (7.3983, 32.6373) (7.3655, 32.5606) (7.3332, 32.4838) (7.3017, 32.4067) (7.2716, 32.3292) (7.244, 32.251) (7.2245, 32.1878) (7.2117, 32.1398) (7.204, 32.1076) (7.2004, 32.0914) knots -1 -1 -1 -1 -1 -1 -0.98571429 -0.97142857 -0.95714286 -0.94285714 -0.92857143 -0.91428571 -0.9 -0.88571429 -0.87142857 -0.85714286 -0.84285714 -0.82857143 -0.81428571 -0.8 -0.78571429 -0.77142857 -0.75714286 -0.74285714 -0.72857143 -0.71428571 -0.7 -0.68571429 -0.67142857 -0.65714286 -0.64285714 -0.62857143 -0.61428571 -0.6 -0.58571429 -0.57142857 -0.55714286 -0.54285714 -0.52857143 -0.51428571 -0.5 -0.48571429 -0.47142857 -0.45714286 -0.44285714 -0.42857143 -0.41428571 -0.4 -0.38571429 -0.37142857 -0.35714286 -0.34285714 -0.32857143 -0.31428571 -0.3 -0.28571429 -0.27142857 -0.25714286 -0.24285714 -0.22857143 -0.21428571 -0.2 -0.18571429 -0.17142857 -0.15714286 -0.14285714 -0.12857143 -0.11428571 -0.1 -0.08571429 -0.07142857 -0.05714286 -0.04285714 -0.02857143 -0.01428571 0 0 0 0 0 0
  line L29 (7.2004, 32.0914) -> (7.0705, 31.5136)
  arc A59 (5.2505, 30.2976) -> (7.0705, 31.5136) centre (5.5216, 31.8618) ccw
  arc A60 (5.2505, 30.2976) -> (4.3689, 30.4372) centre (0, 0) ccw
  arc A61 (3.0138, 32.1561) -> (4.3689, 30.4372) centre (4.5945, 32.0086) ccw
  line L30 (3.0138, 32.1561) -> (3.0688, 32.7458)
  spline S30 degree 5 poles (3.0688, 32.7458) (3.0704, 32.7623) (3.073, 32.7953) (3.0757, 32.8449) (3.0767, 32.9111) (3.0745, 32.994) (3.0699, 33.0769) (3.0638, 33.16) (3.0568, 33.2431) (3.0493, 33.3262) (3.0411, 33.4093) (3.0322, 33.4924) (3.0223, 33.5756) (3.0111, 33.6587) (2.9988, 33.7419) (2.9854, 33.825) (2.971, 33.9081) (2.9558, 33.9913) (2.9399, 34.0744) (2.9233, 34.1575) (2.9061, 34.2405) (2.8882, 34.3236) (2.8696, 34.4066) (2.8502, 34.4896) (2.8301, 34.5725) (2.8093, 34.6554) (2.7878, 34.7383) (2.7657, 34.8211) (2.7429, 34.9039) (2.7195, 34.9867) (2.6956, 35.0694) (2.671, 35.152) (2.6459, 35.2346) (2.6201, 35.3172) (2.5937, 35.3997) (2.5668, 35.4821) (2.5393, 35.5645) (2.5113, 35.6469) (2.4827, 35.7291) (2.4535, 35.8113) (2.4238, 35.8935) (2.3936, 35.9756) (2.3629, 36.0576) (2.3316, 36.1395) (2.2998, 36.2214) (2.2675, 36.3032) (2.2347, 36.385) (2.2013, 36.4666) (2.1675, 36.5482) (2.1332, 36.6297) (2.0984, 36.7112) (2.0631, 36.7925) (2.0274, 36.8738) (1.9911, 36.955) (1.9544, 37.0361) (1.9172, 37.1172) (1.8795, 37.1981) (1.8414, 37.279) (1.8028, 37.3598) (1.7638, 37.4405) (1.7243, 37.5211) (1.6843, 37.6016) (1.6439, 37.682) (1.6031, 37.7623) (1.5618, 37.8425) (1.5201, 37.9227) (1.4779, 38.0027) (1.4353, 38.0826) (1.3923, 38.1625) (1.3489, 38.2422) (1.305, 38.3218) (1.2695, 38.3855) (1.2428, 38.4332) (1.2248, 38.4649) (1.2158, 38.4808) knots 0 0 0 0 0 0 0.01428571 0.02857143 0.04285714 0.05714286 0.07142857 0.08571429 0.1 0.11428571 0.12857143 0.14285714 0.15714286 0.17142857 0.18571429 0.2 0.21428571 0.22857143 0.24285714 0.25714286 0.27142857 0.28571429 0.3 0.31428571 0.32857143 0.34285714 0.35714286 0.37142857 0.38571429 0.4 0.41428571 0.42857143 0.44285714 0.45714286 0.47142857 0.48571429 0.5 0.51428571 0.52857143 0.54285714 0.55714286 0.57142857 0.58571429 0.6 0.61428571 0.62857143 0.64285714 0.65714286 0.67142857 0.68571429 0.7 0.71428571 0.72857143 0.74285714 0.75714286 0.77142857 0.78571429 0.8 0.81428571 0.82857143 0.84285714 0.85714286 0.87142857 0.88571429 0.9 0.91428571 0.92857143 0.94285714 0.95714286 0.97142857 0.98571429 1 1 1 1 1 1
  arc A62 (1.2158, 38.4808) -> (-1.2158, 38.4808) centre (0, 0) ccw
  spline S31 degree 5 poles (-1.2158, 38.4808) (-1.2248, 38.4649) (-1.2428, 38.4332) (-1.2695, 38.3855) (-1.305, 38.3218) (-1.3489, 38.2422) (-1.3923, 38.1625) (-1.4353, 38.0826) (-1.4779, 38.0027) (-1.5201, 37.9227) (-1.5618, 37.8425) (-1.6031, 37.7623) (-1.6439, 37.682) (-1.6843, 37.6016) (-1.7243, 37.5211) (-1.7638, 37.4405) (-1.8028, 37.3598) (-1.8414, 37.279) (-1.8795, 37.1981) (-1.9172, 37.1172) (-1.9544, 37.0361) (-1.9911, 36.955) (-2.0274, 36.8738) (-2.0631, 36.7925) (-2.0984, 36.7112) (-2.1332, 36.6297) (-2.1675, 36.5482) (-2.2013, 36.4666) (-2.2347, 36.385) (-2.2675, 36.3032) (-2.2998, 36.2214) (-2.3316, 36.1395) (-2.3629, 36.0576) (-2.3936, 35.9756) (-2.4238, 35.8935) (-2.4535, 35.8113) (-2.4827, 35.7291) (-2.5113, 35.6469) (-2.5393, 35.5645) (-2.5668, 35.4821) (-2.5937, 35.3997) (-2.6201, 35.3172) (-2.6459, 35.2346) (-2.671, 35.152) (-2.6956, 35.0694) (-2.7195, 34.9867) (-2.7429, 34.9039) (-2.7657, 34.8211) (-2.7878, 34.7383) (-2.8093, 34.6554) (-2.8301, 34.5725) (-2.8502, 34.4896) (-2.8696, 34.4066) (-2.8882, 34.3236) (-2.9061, 34.2405) (-2.9233, 34.1575) (-2.9399, 34.0744) (-2.9558, 33.9913) (-2.971, 33.9081) (-2.9854, 33.825) (-2.9988, 33.7419) (-3.0111, 33.6587) (-3.0223, 33.5756) (-3.0322, 33.4924) (-3.0411, 33.4093) (-3.0493, 33.3262) (-3.0568, 33.2431) (-3.0638, 33.16) (-3.0699, 33.0769) (-3.0745, 32.994) (-3.0767, 32.9111) (-3.0757, 32.8449) (-3.073, 32.7953) (-3.0704, 32.7623) (-3.0688, 32.7458) knots -1 -1 -1 -1 -1 -1 -0.98571429 -0.97142857 -0.95714286 -0.94285714 -0.92857143 -0.91428571 -0.9 -0.88571429 -0.87142857 -0.85714286 -0.84285714 -0.82857143 -0.81428571 -0.8 -0.78571429 -0.77142857 -0.75714286 -0.74285714 -0.72857143 -0.71428571 -0.7 -0.68571429 -0.67142857 -0.65714286 -0.64285714 -0.62857143 -0.61428571 -0.6 -0.58571429 -0.57142857 -0.55714286 -0.54285714 -0.52857143 -0.51428571 -0.5 -0.48571429 -0.47142857 -0.45714286 -0.44285714 -0.42857143 -0.41428571 -0.4 -0.38571429 -0.37142857 -0.35714286 -0.34285714 -0.32857143 -0.31428571 -0.3 -0.28571429 -0.27142857 -0.25714286 -0.24285714 -0.22857143 -0.21428571 -0.2 -0.18571429 -0.17142857 -0.15714286 -0.14285714 -0.12857143 -0.11428571 -0.1 -0.08571429 -0.07142857 -0.05714286 -0.04285714 -0.02857143 -0.01428571 0 0 0 0 0 0
  line L31 (-3.0688, 32.7458) -> (-3.0138, 32.1561)
  arc A63 (-4.3689, 30.4372) -> (-3.0138, 32.1561) centre (-4.5945, 32.0086) ccw
  arc A64 (-4.3689, 30.4372) -> (-5.2505, 30.2976) centre (0, 0) ccw
  arc A65 (-7.0705, 31.5136) -> (-5.2505, 30.2976) centre (-5.5216, 31.8618) ccw
  line L32 (-7.0705, 31.5136) -> (-7.2004, 32.0914)
  spline S32 degree 5 poles (-7.2004, 32.0914) (-7.204, 32.1076) (-7.2117, 32.1398) (-7.2245, 32.1878) (-7.244, 32.251) (-7.2716, 32.3292) (-7.3017, 32.4067) (-7.3332, 32.4838) (-7.3655, 32.5606) (-7.3983, 32.6373) (-7.4318, 32.7139) (-7.4659, 32.7902) (-7.5011, 32.8662) (-7.5373, 32.9418) (-7.5748, 33.0171) (-7.6133, 33.092) (-7.6526, 33.1666) (-7.6928, 33.241) (-7.7336, 33.3151) (-7.775, 33.389) (-7.817, 33.4627) (-7.8597, 33.5362) (-7.9031, 33.6094) (-7.9471, 33.6823) (-7.9919, 33.755) (-8.0373, 33.8274) (-8.0834, 33.8996) (-8.13, 33.9715) (-8.1773, 34.0432) (-8.225, 34.1147) (-8.2734, 34.1859) (-8.3223, 34.257) (-8.3717, 34.3277) (-8.4218, 34.3983) (-8.4723, 34.4686) (-8.5234, 34.5387) (-8.575, 34.6086) (-8.6271, 34.6782) (-8.6798, 34.7476) (-8.7329, 34.8168) (-8.7865, 34.8857) (-8.8406, 34.9545) (-8.8952, 35.023) (-8.9503, 35.0912) (-9.0058, 35.1593) (-9.0618, 35.2271) (-9.1183, 35.2947) (-9.1752, 35.3621) (-9.2326, 35.4292) (-9.2904, 35.4962) (-9.3487, 35.5629) (-9.4074, 35.6293) (-9.4665, 35.6956) (-9.5261, 35.7616) (-9.5861, 35.8274) (-9.6465, 35.893) (-9.7073, 35.9583) (-9.7686, 36.0235) (-9.8302, 36.0883) (-9.8923, 36.153) (-9.9548, 36.2175) (-10.0176, 36.2817) (-10.0809, 36.3457) (-10.1446, 36.4095) (-10.2086, 36.473) (-10.2731, 36.5363) (-10.3379, 36.5994) (-10.4031, 36.6623) (-10.4687, 36.7249) (-10.5347, 36.7873) (-10.601, 36.8495) (-10.6544, 36.8991) (-10.6946, 36.9361) (-10.7214, 36.9608) (-10.7349, 36.9731) knots 0 0 0 0 0 0 0.01428571 0.02857143 0.04285714 0.05714286 0.07142857 0.08571429 0.1 0.11428571 0.12857143 0.14285714 0.15714286 0.17142857 0.18571429 0.2 0.21428571 0.22857143 0.24285714 0.25714286 0.27142857 0.28571429 0.3 0.31428571 0.32857143 0.34285714 0.35714286 0.37142857 0.38571429 0.4 0.41428571 0.42857143 0.44285714 0.45714286 0.47142857 0.48571429 0.5 0.51428571 0.52857143 0.54285714 0.55714286 0.57142857 0.58571429 0.6 0.61428571 0.62857143 0.64285714 0.65714286 0.67142857 0.68571429 0.7 0.71428571 0.72857143 0.74285714 0.75714286 0.77142857 0.78571429 0.8 0.81428571 0.82857143 0.84285714 0.85714286 0.87142857 0.88571429 0.9 0.91428571 0.92857143 0.94285714 0.95714286 0.97142857 0.98571429 1 1 1 1 1 1
  arc A66 (-10.7349, 36.9731) -> (-13.0476, 36.2217) centre (0, 0) ccw
  spline S33 degree 5 poles (-13.0476, 36.2217) (-13.0512, 36.2038) (-13.0584, 36.1681) (-13.0692, 36.1145) (-13.0832, 36.043) (-13.1003, 35.9537) (-13.117, 35.8644) (-13.1333, 35.7752) (-13.1491, 35.686) (-13.1644, 35.5969) (-13.1793, 35.5078) (-13.1938, 35.4187) (-13.2078, 35.3297) (-13.2214, 35.2407) (-13.2345, 35.1518) (-13.2472, 35.063) (-13.2594, 34.9741) (-13.2711, 34.8854) (-13.2824, 34.7967) (-13.2932, 34.7081) (-13.3035, 34.6195) (-13.3134, 34.531) (-13.3228, 34.4426) (-13.3317, 34.3542) (-13.3401, 34.266) (-13.348, 34.1778) (-13.3555, 34.0896) (-13.3624, 34.0016) (-13.3689, 33.9136) (-13.3748, 33.8257) (-13.3803, 33.7379) (-13.3852, 33.6502) (-13.3896, 33.5626) (-13.3935, 33.4751) (-13.3969, 33.3877) (-13.3997, 33.3004) (-13.4021, 33.2132) (-13.4038, 33.1262) (-13.4051, 33.0392) (-13.4058, 32.9523) (-13.4059, 32.8656) (-13.4055, 32.779) (-13.4045, 32.6925) (-13.4029, 32.6062) (-13.4007, 32.52) (-13.3979, 32.4339) (-13.3946, 32.348) (-13.3906, 32.2622) (-13.3861, 32.1766) (-13.3809, 32.0911) (-13.3751, 32.0059) (-13.3686, 31.9208) (-13.3614, 31.8359) (-13.3534, 31.7511) (-13.3448, 31.6666) (-13.3355, 31.5823) (-13.3255, 31.4982) (-13.315, 31.4142) (-13.3037, 31.3305) (-13.2917, 31.247) (-13.2788, 31.1637) (-13.2649, 31.0808) (-13.2498, 30.9983) (-13.2335, 30.9162) (-13.2163, 30.8344) (-13.1984, 30.7528) (-13.1798, 30.6714) (-13.1608, 30.5903) (-13.141, 30.5094) (-13.1197, 30.429) (-13.0962, 30.3496) (-13.0748, 30.2869) (-13.0569, 30.2406) (-13.0442, 30.21) (-13.0376, 30.1947) knots -1 -1 -1 -1 -1 -1 -0.98571429 -0.97142857 -0.95714286 -0.94285714 -0.92857143 -0.91428571 -0.9 -0.88571429 -0.87142857 -0.85714286 -0.84285714 -0.82857143 -0.81428571 -0.8 -0.78571429 -0.77142857 -0.75714286 -0.74285714 -0.72857143 -0.71428571 -0.7 -0.68571429 -0.67142857 -0.65714286 -0.64285714 -0.62857143 -0.61428571 -0.6 -0.58571429 -0.57142857 -0.55714286 -0.54285714 -0.52857143 -0.51428571 -0.5 -0.48571429 -0.47142857 -0.45714286 -0.44285714 -0.42857143 -0.41428571 -0.4 -0.38571429 -0.37142857 -0.35714286 -0.34285714 -0.32857143 -0.31428571 -0.3 -0.28571429 -0.27142857 -0.25714286 -0.24285714 -0.22857143 -0.21428571 -0.2 -0.18571429 -0.17142857 -0.15714286 -0.14285714 -0.12857143 -0.11428571 -0.1 -0.08571429 -0.07142857 -0.05714286 -0.04285714 -0.02857143 -0.01428571 0 0 0 0 0 0
  line L33 (-13.0376, 30.1947) -> (-12.8031, 29.6509)
  arc A67 (-13.5607, 27.5975) -> (-12.8031, 29.6509) centre (-14.2608, 29.0223) ccw
  arc A68 (-13.5607, 27.5975) -> (-14.356, 27.1922) centre (0, 0) ccw
  arc A69 (-16.4626, 27.7863) -> (-14.356, 27.1922) centre (-15.0972, 28.5961) ccw
  line L34 (-16.4626, 27.7863) -> (-16.7647, 28.2957)
  spline S34 degree 5 poles (-16.7647, 28.2957) (-16.7732, 28.3099) (-16.7905, 28.3382) (-16.8175, 28.3799) (-16.8556, 28.434) (-16.906, 28.4998) (-16.9585, 28.5642) (-17.0123, 28.6278) (-17.0668, 28.6909) (-17.1217, 28.7537) (-17.1772, 28.8162) (-17.2332, 28.8782) (-17.2901, 28.9396) (-17.348, 29.0004) (-17.4069, 29.0604) (-17.4666, 29.1198) (-17.5272, 29.1786) (-17.5883, 29.2369) (-17.65, 29.2948) (-17.7122, 29.3523) (-17.775, 29.4094) (-17.8383, 29.466) (-17.9021, 29.5222) (-17.9666, 29.578) (-18.0316, 29.6333) (-18.0972, 29.6881) (-18.1633, 29.7425) (-18.2299, 29.7965) (-18.297, 29.8501) (-18.3645, 29.9033) (-18.4325, 29.9561) (-18.5009, 30.0086) (-18.5699, 30.0606) (-18.6392, 30.1123) (-18.709, 30.1635) (-18.7793, 30.2144) (-18.85, 30.2649) (-18.921, 30.315) (-18.9925, 30.3647) (-19.0645, 30.4141) (-19.1368, 30.4631) (-19.2094, 30.5118) (-19.2825, 30.5601) (-19.356, 30.608) (-19.4299, 30.6555) (-19.5041, 30.7027) (-19.5787, 30.7496) (-19.6536, 30.796) (-19.7289, 30.8422) (-19.8046, 30.888) (-19.8806, 30.9334) (-19.957, 30.9785) (-20.0337, 31.0232) (-20.1108, 31.0676) (-20.1882, 31.1116) (-20.2659, 31.1553) (-20.3439, 31.1987) (-20.4223, 31.2417) (-20.501, 31.2844) (-20.58, 31.3267) (-20.6594, 31.3687) (-20.739, 31.4103) (-20.8189, 31.4516) (-20.8992, 31.4926) (-20.9798, 31.5333) (-21.0606, 31.5736) (-21.1418, 31.6135) (-21.2232, 31.6532) (-21.3049, 31.6925) (-21.387, 31.7314) (-21.4693, 31.7701) (-21.5353, 31.8007) (-21.585, 31.8236) (-21.6182, 31.8387) (-21.6348, 31.8463) knots 0 0 0 0 0 0 0.01428571 0.02857143 0.04285714 0.05714286 0.07142857 0.08571429 0.1 0.11428571 0.12857143 0.14285714 0.15714286 0.17142857 0.18571429 0.2 0.21428571 0.22857143 0.24285714 0.25714286 0.27142857 0.28571429 0.3 0.31428571 0.32857143 0.34285714 0.35714286 0.37142857 0.38571429 0.4 0.41428571 0.42857143 0.44285714 0.45714286 0.47142857 0.48571429 0.5 0.51428571 0.52857143 0.54285714 0.55714286 0.57142857 0.58571429 0.6 0.61428571 0.62857143 0.64285714 0.65714286 0.67142857 0.68571429 0.7 0.71428571 0.72857143 0.74285714 0.75714286 0.77142857 0.78571429 0.8 0.81428571 0.82857143 0.84285714 0.85714286 0.87142857 0.88571429 0.9 0.91428571 0.92857143 0.94285714 0.95714286 0.97142857 0.98571429 1 1 1 1 1 1
  arc A70 (-21.6348, 31.8463) -> (-23.6021, 30.417) centre (0, 0) ccw
  spline S35 degree 5 poles (-23.6021, 30.417) (-23.6, 30.3988) (-23.5959, 30.3626) (-23.5895, 30.3083) (-23.5808, 30.236) (-23.5695, 30.1458) (-23.5577, 30.0557) (-23.5456, 29.9658) (-23.5331, 29.8761) (-23.5201, 29.7866) (-23.5068, 29.6972) (-23.493, 29.6081) (-23.4789, 29.5191) (-23.4643, 29.4303) (-23.4493, 29.3417) (-23.4339, 29.2532) (-23.418, 29.165) (-23.4018, 29.077) (-23.3851, 28.9892) (-23.368, 28.9015) (-23.3504, 28.8141) (-23.3325, 28.7269) (-23.3141, 28.6399) (-23.2952, 28.5531) (-23.2759, 28.4666) (-23.2562, 28.3802) (-23.2361, 28.2941) (-23.2155, 28.2082) (-23.1944, 28.1226) (-23.1729, 28.0371) (-23.151, 27.952) (-23.1286, 27.867) (-23.1057, 27.7824) (-23.0824, 27.6979) (-23.0586, 27.6138) (-23.0343, 27.5298) (-23.0096, 27.4462) (-22.9844, 27.3628) (-22.9587, 27.2797) (-22.9325, 27.1969) (-22.9058, 27.1144) (-22.8786, 27.0322) (-22.8509, 26.9502) (-22.8227, 26.8686) (-22.794, 26.7873) (-22.7648, 26.7063) (-22.7351, 26.6256) (-22.7048, 26.5453) (-22.674, 26.4652) (-22.6427, 26.3856) (-22.6108, 26.3062) (-22.5783, 26.2273) (-22.5452, 26.1488) (-22.5115, 26.0707) (-22.4772, 25.993) (-22.4423, 25.9157) (-22.4068, 25.8387) (-22.3708, 25.7622) (-22.3343, 25.686) (-22.297, 25.6103) (-22.259, 25.5351) (-22.2202, 25.4606) (-22.1803, 25.3867) (-22.1395, 25.3136) (-22.0978, 25.2411) (-22.0555, 25.1691) (-22.0128, 25.0975) (-21.9696, 25.0261) (-21.9257, 24.9554) (-21.8807, 24.8855) (-21.8337, 24.8172) (-21.794, 24.7642) (-21.7627, 24.7257) (-21.7412, 24.7005) (-21.7302, 24.6881) knots -1 -1 -1 -1 -1 -1 -0.98571429 -0.97142857 -0.95714286 -0.94285714 -0.92857143 -0.91428571 -0.9 -0.88571429 -0.87142857 -0.85714286 -0.84285714 -0.82857143 -0.81428571 -0.8 -0.78571429 -0.77142857 -0.75714286 -0.74285714 -0.72857143 -0.71428571 -0.7 -0.68571429 -0.67142857 -0.65714286 -0.64285714 -0.62857143 -0.61428571 -0.6 -0.58571429 -0.57142857 -0.55714286 -0.54285714 -0.52857143 -0.51428571 -0.5 -0.48571429 -0.47142857 -0.45714286 -0.44285714 -0.42857143 -0.41428571 -0.4 -0.38571429 -0.37142857 -0.35714286 -0.34285714 -0.32857143 -0.31428571 -0.3 -0.28571429 -0.27142857 -0.25714286 -0.24285714 -0.22857143 -0.21428571 -0.2 -0.18571429 -0.17142857 -0.15714286 -0.14285714 -0.12857143 -0.11428571 -0.1 -0.08571429 -0.07142857 -0.05714286 -0.04285714 -0.02857143 -0.01428571 0 0 0 0 0 0
  line L35 (-21.7302, 24.6881) -> (-21.3391, 24.2433)
  arc A71 (-21.4251, 22.0563) -> (-21.3391, 24.2433) centre (-22.5312, 23.195) ccw
  arc A72 (-21.4251, 22.0563) -> (-22.0563, 21.4251) centre (0, 0) ccw
  arc A73 (-24.2433, 21.3391) -> (-22.0563, 21.4251) centre (-23.195, 22.5312) ccw
  line L36 (-24.2433, 21.3391) -> (-24.6881, 21.7302)
  spline S36 degree 5 poles (-24.6881, 21.7302) (-24.7005, 21.7412) (-24.7257, 21.7627) (-24.7642, 21.794) (-24.8172, 21.8337) (-24.8855, 21.8807) (-24.9554, 21.9257) (-25.0261, 21.9696) (-25.0975, 22.0128) (-25.1691, 22.0555) (-25.2411, 22.0978) (-25.3136, 22.1395) (-25.3867, 22.1803) (-25.4606, 22.2202) (-25.5351, 22.259) (-25.6103, 22.297) (-25.686, 22.3343) (-25.7622, 22.3708) (-25.8387, 22.4068) (-25.9157, 22.4423) (-25.993, 22.4772) (-26.0707, 22.5115) (-26.1488, 22.5452) (-26.2273, 22.5783) (-26.3062, 22.6108) (-26.3856, 22.6427) (-26.4652, 22.674) (-26.5453, 22.7048) (-26.6256, 22.7351) (-26.7063, 22.7648) (-26.7873, 22.794) (-26.8686, 22.8227) (-26.9502, 22.8509) (-27.0322, 22.8786) (-27.1144, 22.9058) (-27.1969, 22.9325) (-27.2797, 22.9587) (-27.3628, 22.9844) (-27.4462, 23.0096) (-27.5298, 23.0343) (-27.6138, 23.0586) (-27.6979, 23.0824) (-27.7824, 23.1057) (-27.867, 23.1286) (-27.952, 23.151) (-28.0371, 23.1729) (-28.1226, 23.1944) (-28.2082, 23.2155) (-28.2941, 23.2361) (-28.3802, 23.2562) (-28.4666, 23.2759) (-28.5531, 23.2952) (-28.6399, 23.3141) (-28.7269, 23.3325) (-28.8141, 23.3504) (-28.9015, 23.368) (-28.9892, 23.3851) (-29.077, 23.4018) (-29.165, 23.418) (-29.2532, 23.4339) (-29.3417, 23.4493) (-29.4303, 23.4643) (-29.5191, 23.4789) (-29.6081, 23.493) (-29.6972, 23.5068) (-29.7866, 23.5201) (-29.8761, 23.5331) (-29.9658, 23.5456) (-30.0557, 23.5577) (-30.1458, 23.5695) (-30.236, 23.5808) (-30.3083, 23.5895) (-30.3626, 23.5959) (-30.3988, 23.6) (-30.417, 23.6021) knots 0 0 0 0 0 0 0.01428571 0.02857143 0.04285714 0.05714286 0.07142857 0.08571429 0.1 0.11428571 0.12857143 0.14285714 0.15714286 0.17142857 0.18571429 0.2 0.21428571 0.22857143 0.24285714 0.25714286 0.27142857 0.28571429 0.3 0.31428571 0.32857143 0.34285714 0.35714286 0.37142857 0.38571429 0.4 0.41428571 0.42857143 0.44285714 0.45714286 0.47142857 0.48571429 0.5 0.51428571 0.52857143 0.54285714 0.55714286 0.57142857 0.58571429 0.6 0.61428571 0.62857143 0.64285714 0.65714286 0.67142857 0.68571429 0.7 0.71428571 0.72857143 0.74285714 0.75714286 0.77142857 0.78571429 0.8 0.81428571 0.82857143 0.84285714 0.85714286 0.87142857 0.88571429 0.9 0.91428571 0.92857143 0.94285714 0.95714286 0.97142857 0.98571429 1 1 1 1 1 1
  arc A74 (-30.417, 23.6021) -> (-31.8463, 21.6348) centre (0, 0) ccw